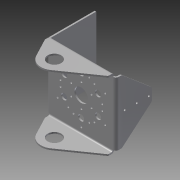
# Autodesk Inventor part: Plate 2 (Back)
Saved by Autodesk Inventor 2014 (Build 180170000, 170)
## iProperties
Created: 2014-01-12
Part Number: Plate 2 (Back)
Material: Steel
Document SubType Name: Sheet Metal
Designer: Andrew Toennies
Density: 7.85 g/cm^3
Sheet Metal Rule: Default
Appearance: Steel
Mass: 842.273 g
Surface Area: 729.034 cm^2
Volume: 107.296 cm^3
Author: Andrew Toennies
Autodesk Inventor part; units mm, degrees
ref_plane "YZ Plane" through (0, 0, 0) normal (1, 0, 0) x (0, 1, 0)
ref_plane "XZ Plane" through (0, 0, 0) normal (0, 1, 0) x (-1, 0, 0)
ref_plane "XY Plane" through (0, 0, 0) normal (0, 0, 1) x (1, 0, 0)
sketch "Sketch1" plane through (0, 0, 0) normal (0, 0, 1) x (1, 0, 0)
  circle A0 centre (0, 0) radius 66.675 construction
  circle A1 centre (0, 0) radius 14.2875
  circle A2 centre (0, 41.275) radius 6.3881
  line L0 (0, 0) -> (0, 41.275) construction
  circle A3 centre (0, 41.275) radius 16.637 construction
  circle A4 centre (0, 57.912) radius 2.3812
  circle A5 centre (16.637, 41.275) radius 2.3812
  circle A6 centre (0, 24.638) radius 2.3812
  circle A7 centre (-16.637, 41.275) radius 2.3813
  line L1 (0, 41.275) -> (0, 57.912) construction
  line L2 (-16.637, 41.275) -> (16.637, 41.275) construction
  circle A8 centre (-50.1533, 28.956) radius 2.3812
  circle A9 centre (-44.0637, 6.2294) radius 2.3813
  circle A10 centre (-35.7452, 20.6375) radius 6.3881
  circle A11 centre (-27.4267, 35.0456) radius 2.3812
  circle A12 centre (-21.3371, 12.319) radius 2.3812
  circle A13 centre (-50.1533, -28.956) radius 2.3812
  circle A14 centre (-27.4267, -35.0456) radius 2.3813
  circle A15 centre (-35.7452, -20.6375) radius 6.3881
  circle A16 centre (-44.0637, -6.2294) radius 2.3812
  circle A17 centre (-21.3371, -12.319) radius 2.3812
  circle A18 centre (0, -57.912) radius 2.3812
  circle A19 centre (16.637, -41.275) radius 2.3813
  circle A20 centre (0, -41.275) radius 6.3881
  circle A21 centre (-16.637, -41.275) radius 2.3812
  circle A22 centre (0, -24.638) radius 2.3812
  circle A23 centre (50.1533, -28.956) radius 2.3812
  circle A24 centre (44.0637, -6.2294) radius 2.3813
  circle A25 centre (35.7452, -20.6375) radius 6.3881
  circle A26 centre (27.4267, -35.0456) radius 2.3812
  circle A27 centre (21.3371, -12.319) radius 2.3812
  circle A28 centre (50.1533, 28.956) radius 2.3812
  circle A29 centre (27.4267, 35.0456) radius 2.3813
  circle A30 centre (35.7452, 20.6375) radius 6.3881
  circle A31 centre (44.0637, 6.2294) radius 2.3812
  circle A32 centre (21.3371, 12.319) radius 2.3812
  line L3 (-66.675, 66.675) -> (66.675, 66.675)
  line L4 (66.675, 66.675) -> (66.675, -66.675)
  line L5 (66.675, -66.675) -> (-66.675, -66.675)
  line L6 (-66.675, -66.675) -> (-66.675, 66.675)
  dimension "d2" = 133.35
  dimension "d3" = 28.575
  dimension "d4" = 12.7762
  dimension "d5" = 41.275
  dimension "d6" = 33.274
  dimension "d7" = 4.7625
  dimension "d8" = 4.7625
  dimension "d9" = 4.7625
  dimension "d10" = 4.7625
  dimension "d11" = 360
  measures "d2" diameter of A0
  measures "d3" diameter of A1
  measures "d4" diameter of A2
  measures "d5" distance of L0.start L0.end
  measures "d6" diameter of A3
  measures "d7" diameter of A4
  measures "d8" diameter of A5
  measures "d9" diameter of A6
  measures "d10" diameter of A7
extrude "Plate1" add sketch "Sketch1" along normal blind 3.175
sketch "Sketch3" plane through (66.675, -69.85, 6.35) normal (0, -1, 0) x (1, 0, 0)
  line L0 (-133.35, 0) -> (0, 0)
  line L1 (0, 0) -> (0, 69.85)
  line L2 (0, 69.85) -> (-133.35, 69.85)
  line L3 (-133.35, 69.85) -> (-133.35, 0)
  constraints: 6 end point, 1 horizontal, 1 perpendicular, 1 vertical
edge flange "Flange2" height 76.2 angle 90 thickness 3.175 bend radius 3.175 thickness toward (0, -1, 0) relief straight relief width 3.175 relief depth 1.5875 corner gap 3.175 corner form 0 edges at (0, -66.675, 3.175) (0, 66.675, 3.175) wall of the first edge with corners at (-66.675, -69.85, 6.35) (66.675, -69.85, 6.35) (66.675, -69.85, 76.2) (-66.675, -69.85, 76.2)
bend "Bend2"
corner "Corner2"
sketch "Sketch5" plane through (-66.675, 69.85, 76.2) normal (0, -1, 0) x (1, 0, 0)
  line L0 (38.7453, -36.6683) -> (41.7281, -43.3665) projected
  line L1 (41.7281, -43.3665) -> (49.0204, -44.1324) projected
  line L2 (49.0204, -44.1324) -> (53.3297, -38.2) projected
  line L3 (53.3297, -38.2) -> (50.3469, -31.5018) projected
  line L4 (50.3469, -31.5018) -> (43.0546, -30.736) projected
  line L5 (43.0546, -30.736) -> (38.7453, -36.6683) projected
  line L6 (53.3297, -38.2) -> (38.7453, -36.6683) construction
  line L7 (49.0204, -44.1324) -> (43.0546, -30.736) construction
  circle A0 centre (46.0375, -37.4342) radius 14.2875
  point P0 (66.675, -76.2)
  dimension "d39" = 28.575
  constraints: 4 end point, 2 midpoint, 2 parallel, 1 centre point
  measures "d39" diameter of A0
extrude "Cut2" cut sketch "Sketch5" against normal mid plane 2540 contours L5 L4 L3 L2 L1 L0 | A0
sketch "Sketch6" plane through (-66.675, 73.025, 76.2) normal (0, 1, 0) x (1, 0, 0)
  circle A0 centre (46.0375, 37.4342) radius 14.2875 projected
  line L0 (133.35, 69.85) -> (0, 69.85) projected
  line L1 (0, 0) -> (0, 69.85) projected
  line L2 (133.35, 0) -> (0, 0) projected
  line L3 (133.35, 69.85) -> (133.35, 0) projected
  arc A1 (20.7582, 24.1116) -> (62.3859, 13.9978) centre (46.0375, 37.4342) ccw
  line L4 (0, 63.5) -> (20.7582, 24.1116)
  line L5 (133.35, 63.5) -> (62.3859, 13.9978)
  point P0 (66.675, 76.2)
  dimension "d42" = 57.15
  dimension "d43" = 6.35
  dimension "d44" = 6.35
  constraints: 4 end point, 2 point on circle, 2 point on line, 2 tangent, 1 centre point, 1 coincident
  measures "d42" diameter of A1
  measures "d43" distance from line of L0 L4.start
  measures "d44" distance of L5.start L0.start
extrude "Cut3" cut sketch "Sketch6" against normal blind 254 contours L3 L2 L1 L4 A1 L5
fillet "Fillet1" radius 3.175 4 edges at (66.675, 71.4375, 12.7) (66.675, -71.4375, 12.7) (-66.675, 71.4375, 12.7) (-66.675, -71.4375, 12.7)
sketch "Sketch7" plane through (69.85, -66.675, -3.175) normal (1, 0, 0) x (0, 1, 0)
  line L0 (133.35, 0) -> (0, 0)
  line L1 (0, 0) -> (0, -69.85)
  line L2 (0, -69.85) -> (133.35, -69.85)
  line L3 (133.35, -69.85) -> (133.35, 0)
  constraints: 6 end point, 1 horizontal, 1 perpendicular, 1 vertical
edge flange "Flange3" height 76.2 angle 90 thickness 3.175 bend radius 3.175 thickness toward (1, 0, 0) relief straight relief width 3.175 relief depth 1.5875 edges at (66.675, 0, 0) wall of the first edge with corners at (69.85, 66.675, -3.175) (69.85, -66.675, -3.175) (69.85, -66.675, -73.025) (69.85, 66.675, -73.025)
bend "Bend3"
corner "Corner3"
sketch "Sketch8" plane through (69.85, -66.675, -73.025) normal (-1, 0, 0) x (0, 0, 1)
  line L0 (0, 133.35) -> (69.85, 133.35) projected
  line L1 (0, 133.35) -> (0, 0) projected
  line L2 (0, 0) -> (69.85, 0) projected
  line L3 (0, 79.375) -> (63.5, 133.35)
  line L4 (0, 53.975) -> (63.5, 0)
  point P0 (73.025, 66.675)
  dimension "d58" = 25.4
  dimension "d59" = 53.975
  dimension "d60" = 6.35
  dimension "d61" = 6.35
  constraints: 4 end point, 4 point on line
  measures "d58" distance of L4.start L3.start
  measures "d59" distance from line of L2 L4.start
  measures "d60" distance of L0.end L3.end
  measures "d61" distance of L2.end L4.end
extrude "Cut4" cut sketch "Sketch8" against normal blind 3.175
fillet "Fillet2" radius 6.35 4 edges at (71.4375, -66.675, -9.525) (71.4375, -12.7, -73.025) (71.4375, 12.7, -73.025) (71.4375, 66.675, -9.525)
sketch "Sketch9" plane through (69.85, -66.675, -3.175) normal (-1, 0, 0) x (0, 0, 1)
  arc A0 (-61.4313, 66.7512) -> (-65.5687, 66.7512) centre (-63.5, 66.675) ccw projected
  arc A1 (-36.0313, 66.7512) -> (-40.1687, 66.7512) centre (-38.1, 66.675) ccw projected
  arc A2 (-10.6313, 66.7512) -> (-14.7687, 66.7512) centre (-12.7, 66.675) ccw projected
  circle A3 centre (-63.5, 66.675) radius 2.0828
  circle A4 centre (-38.1, 66.675) radius 2.0828
  circle A5 centre (-12.7, 66.675) radius 2.0828
  point P0 (3.175, 66.675)
  dimension "d65" = 4.1656
  dimension "d66" = 4.1656
  dimension "d67" = 4.1656
  constraints: 3 centre point, 3 coincident
  measures "d65" diameter of A3
  measures "d66" diameter of A4
  measures "d67" diameter of A5
extrude "Cut5" cut sketch "Sketch9" against normal blind 3.175
sketch "Sketch11" plane through (-69.85, 66.675, -3.175) normal (-1, 0, 0) x (0, -1, 0)
  line L0 (133.35, 0) -> (0, 0)
  line L1 (0, 0) -> (0, -95.25)
  line L2 (0, -95.25) -> (133.35, -95.25)
  line L3 (133.35, -95.25) -> (133.35, 0)
  constraints: 6 end point, 1 horizontal, 1 perpendicular, 1 vertical
edge flange "Flange4" height 101.6 angle 90 thickness 3.175 bend radius 3.175 thickness toward (-1, 0, 0) relief straight relief width 3.175 relief depth 1.5875 edges at (-66.675, 0, 0) wall of the first edge with corners at (-69.85, -66.675, -3.175) (-69.85, 66.675, -3.175) (-69.85, 66.675, -98.425) (-69.85, -66.675, -98.425)
bend "Bend4"
corner "Corner4"
equation "\"d62\" = Thickness"
equation "\"d68\" = Thickness"
equation "\"d23\" = BendReliefWidth"
equation "\"d24\" = BendReliefDepth"
equation "\"d25\" = MinimumRemnant"
equation "\"d26\" = BendRadius"
equation "\"d30\" = CornerReliefSize"
equation "\"d31\" = GapSize"
equation "\"d32\" = JacobiRadiusSize"
equation "\"d48\" = BendReliefWidth"
equation "\"d49\" = BendReliefDepth"
equation "\"d50\" = MinimumRemnant"
equation "\"d51\" = BendRadius"
equation "\"d54\" = BendRadius"
equation "\"d55\" = CornerReliefSize"
equation "\"d56\" = GapSize"
equation "\"d57\" = JacobiRadiusSize"
equation "\"d71\" = BendReliefWidth"
equation "\"d72\" = BendReliefDepth"
equation "\"d73\" = MinimumRemnant"
equation "\"d74\" = BendRadius"
equation "\"d77\" = BendRadius"
equation "\"d78\" = CornerReliefSize"
equation "\"d79\" = GapSize"
equation "\"d80\" = JacobiRadiusSize"
equation "\"BendRadius\" = Thickness"
equation "\"BendReliefWidth\" = Thickness"
equation "\"BendReliefDepth\" = 0.5 * Thickness"
equation "\"CornerReliefSize\" = 4 * Thickness"
equation "\"MinimumRemnant\" = 2 * Thickness"
equation "\"TransitionRadius\" = BendRadius"
equation "\"JacobiRadiusSize\" = BendRadius"
equation "\"GapSize\" = Thickness"
equation "\"d12\" = BendRadius"
equation "\"Thickness\" = 3.175"
body "Solid1"
